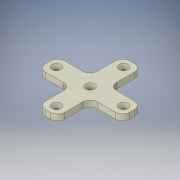
# Autodesk Inventor part: plus sign
Saved by Autodesk Inventor 2016 (Build 200138000, 138)
## iProperties
Created: 2017-03-27
Part Number: plus sign
Material: Polypropylene
Document SubType Name: Modeling
Designer: jwillauer
Density: 0.899 g/cm^3
Appearance: Smooth - Ivory
Author: jwillauer
Autodesk Inventor part; units mm, degrees
ref_plane "YZ Plane" through (0, 0, 0) normal (1, 0, 0) x (0, 1, 0)
ref_plane "XZ Plane" through (0, 0, 0) normal (0, 1, 0) x (-1, 0, 0)
ref_plane "XY Plane" through (0, 0, 0) normal (0, 0, 1) x (1, 0, 0)
sketch "Sketch1" plane through (0, 0, 0) normal (0, 1, 0) x (-1, 0, 0)
  line L0 (0, -23.3395) -> (-88.9, -23.3395)
  line L1 (-88.9, -23.3395) -> (-88.9, 65.5605)
  line L2 (-88.9, 65.5605) -> (0, 65.5605)
  line L3 (0, 65.5605) -> (0, -23.3395)
  point P0 (0, 0)
  dimension "d0" = 88.9
  dimension "d1" = 88.9
  constraints: 8 end point, 2 parallel, 1 horizontal, 1 perpendicular
  measures "d0" distance between parallel lines of L1 L3
  measures "d1" distance between parallel lines of L2 L0
extrude "Extrusion1" add sketch "Sketch1" along normal blind 6.35
sketch "Sketch2" plane through (0, 6.35, 0) normal (0, 1, 0) x (1, 0, 0)
  line L0 (88.9, -65.5605) -> (88.9, 23.3395) projected
  line L1 (88.9, 23.3395) -> (0, 23.3395) projected
  point P0 (0, 0)
  point P1 (44.45, -21.1105)
  point P2 (80.01, -21.1105)
  point P3 (8.89, -21.1105)
  point P4 (44.45, 14.4495)
  point P5 (44.45, -56.6705)
  dimension "d4" = 44.45
  dimension "d5" = 44.45
  dimension "d6" = 35.56
  dimension "d7" = 35.56
  dimension "d8" = 35.56
  dimension "d9" = 35.56
  measures "d4" distance from line of L0 point (44.45, -21.11)
  measures "d5" distance from line of L1 point (44.45, -21.11)
  measures "d6" distance of point (80.01, -21.11) point (44.45, -21.11)
  measures "d7" distance of point (44.45, -21.11) point (44.45, 14.45)
  measures "d8" distance of point (44.45, -21.11) point (8.89, -21.11)
  measures "d9" distance of point (44.45, -21.11) point (44.45, -56.67)
hole "Hole1" at (44.45, 6.35, 21.1105) at (80.01, 6.35, 21.1105) at (8.89, 6.35, 21.1105) at (44.45, 6.35, -14.4495) at (44.45, 6.35, 56.6705) direction (0, -1, 0) diameter 3.556 end through all countersink diameter 9.525 countersink angle 82
sketch "Sketch3" plane through (0, 6.35, 0) normal (0, 1, 0) x (1, 0, 0)
  line L0 (88.9, 23.3395) -> (0, 23.3395) projected
  line L1 (88.9, -65.5605) -> (0, -65.5605) projected
  line L2 (0, -65.5605) -> (0, 23.3395) projected
  line L3 (88.9, 23.3395) -> (88.9, -65.5605) projected
  line L4 (34.29, 15.7195) -> (34.29, -3.3305)
  line L5 (34.29, -38.8905) -> (34.29, -57.9405)
  line L6 (54.61, 15.7195) -> (54.61, -3.3305)
  line L7 (54.61, -38.8905) -> (54.61, -57.9405)
  line L8 (7.62, -31.2705) -> (26.67, -31.2705)
  line L9 (62.23, -31.2705) -> (81.28, -31.2705)
  line L10 (7.62, -10.9505) -> (26.67, -10.9505)
  line L11 (62.23, -10.9505) -> (81.28, -10.9505)
  line L12 (0, -18.5705) -> (0, -23.6505)
  line L13 (41.91, -65.5605) -> (46.99, -65.5605)
  line L14 (88.9, -23.6505) -> (88.9, -18.5705)
  line L15 (41.91, 23.3395) -> (46.99, 23.3395)
  arc A0 (41.91, 23.3395) -> (34.29, 15.7195) centre (41.91, 15.7195) ccw
  arc A1 (54.61, 15.7195) -> (46.99, 23.3395) centre (46.99, 15.7195) ccw
  arc A2 (26.67, -10.9505) -> (34.29, -3.3305) centre (26.67, -3.3305) ccw
  arc A3 (7.62, -10.9505) -> (0, -18.5705) centre (7.62, -18.5705) ccw
  arc A4 (0, -23.6505) -> (7.62, -31.2705) centre (7.62, -23.6505) ccw
  arc A5 (34.29, -38.8905) -> (26.67, -31.2705) centre (26.67, -38.8905) ccw
  arc A6 (34.29, -57.9405) -> (41.91, -65.5605) centre (41.91, -57.9405) ccw
  arc A7 (46.99, -65.5605) -> (54.61, -57.9405) centre (46.99, -57.9405) ccw
  arc A8 (62.23, -31.2705) -> (54.61, -38.8905) centre (62.23, -38.8905) ccw
  arc A9 (81.28, -31.2705) -> (88.9, -23.6505) centre (81.28, -23.6505) ccw
  arc A10 (88.9, -18.5705) -> (81.28, -10.9505) centre (81.28, -18.5705) ccw
  arc A11 (54.61, -3.3305) -> (62.23, -10.9505) centre (62.23, -3.3305) ccw
  point P0 (0, 0)
  dimension "d21" = 7.62
  constraints: 24 end point, 24 point on circle, 24 tangent, 12 centre point, 11 equal radius, 3 collinear, 1 vertical
  measures "d21" radius of A0
extrude "Extrusion2" cut sketch "Sketch3" against normal blind 6.35 contours L3 A10 L11 A11 L6 A1 L0 | A0 L4 A2 L10 A3 L2 L0 | L3 L1 A7 L7 A8 L9 A9 | A4 L8 A5 L5 A6 L1 L2
equation "\"d4\" = 0.5 * d1"
equation "\"d5\" = 0.5 * d1"
body "Solid1"
